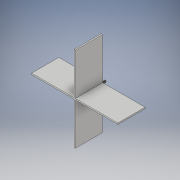
# Autodesk Inventor part: servo part1
Saved by Autodesk Inventor 2019 (Build 230136000, 136)
## iProperties
Created: 2020-02-19
Part Number: servo part1
Material: Generic
Document SubType Name: Modeling
Designer: LENOVO
Density: 1 g/cm^3
Appearance: Default
Author: LENOVO
Autodesk Inventor part; units mm, degrees
ref_plane "YZ Plane" through (0, 0, 0) normal (1, 0, 0) x (0, 1, 0)
ref_plane "XZ Plane" through (0, 0, 0) normal (0, 1, 0) x (-1, 0, 0)
ref_plane "XY Plane" through (0, 0, 0) normal (0, 0, 1) x (1, 0, 0)
sketch "Sketch1" plane through (0, 0, 0) normal (0, 0, 1) x (1, 0, 0)
  circle A0 centre (0, 0) radius 1.5
  dimension "d0" = 3
  constraints: 1 centre point, 1 coincident
  measures "d0" diameter of A0
extrude "Extrusion1" add sketch "Sketch1" along normal blind 4
sketch "Sketch2" plane through (0, 0, 4) normal (0, 0, 1) x (1, 0, 0)
  line L0 (1, 0) -> (-1, 0)
  line L1 (-1, 0) -> (-1, -4)
  line L2 (-1, -4) -> (1, -4)
  line L3 (1, -4) -> (1, 0)
  line L4 (1, 0) -> (-1, 0)
  line L5 (-1, 0) -> (-1, 4)
  line L6 (-1, 4) -> (1, 4)
  line L7 (1, 4) -> (1, 0)
  point P0 (0, 0)
  dimension "d3" = 2
  dimension "d4" = 4
  dimension "d5" = 4
  constraints: 16 end point, 4 parallel, 2 horizontal, 2 perpendicular, 1 point on line
  measures "d3" distance of L2.end L1.end
  measures "d4" distance of L1.end L0.end
  measures "d5" distance of L4.end L5.end
extrude "Extrusion2" add sketch "Sketch2" along normal blind 2
sketch "Sketch3" plane through (0, 0, 4) normal (0, 0, 1) x (1, 0, 0)
  line L0 (1, -4) -> (1, 4) projected
  line L1 (1, 1) -> (5, 1)
  line L2 (5, 1) -> (5, -1)
  line L3 (5, -1) -> (1, -1)
  line L4 (1, -1) -> (1, 1)
  line L5 (-1, 4) -> (-1, -4) projected
  line L6 (-1, 1) -> (-5, 1)
  line L7 (-5, 1) -> (-5, -1)
  line L8 (-5, -1) -> (-1, -1)
  line L9 (-1, -1) -> (-1, 1)
  point P0 (0, 0)
  dimension "d8" = 4
  dimension "d9" = 2
  dimension "d10" = 4
  constraints: 16 end point, 4 parallel, 2 horizontal, 2 perpendicular, 2 point on line
  measures "d8" distance of L2.end L3.end
  measures "d9" distance of L1.end L2.end
  measures "d10" distance of L8.end L7.end
extrude "Extrusion3" add sketch "Sketch3" along normal blind 2
sketch "Sketch4" plane through (0, 0, 4) normal (0, 0, -1) x (-1, 0, 0)
  line L0 (-5, 1) -> (-5, -1) projected
  line L1 (-1.118, 1) -> (-5, 1) projected
  line L2 (-5, -1) -> (-1.5, -1)
  line L3 (-1.5, -1) -> (-1.5, 1)
  line L4 (-1.5, 1) -> (-5, 1)
  line L5 (-5, 1) -> (-5, -1)
  line L6 (1, 4) -> (1, 1.118) projected
  line L7 (-1, 1.118) -> (-1, 4) projected
  line L8 (1, 4) -> (-1, 4)
  line L9 (-1, 4) -> (-1, 1.5)
  line L10 (-1, 1.5) -> (1, 1.5)
  line L11 (1, 1.5) -> (1, 4)
  line L12 (5, -1) -> (1, -1) projected
  line L13 (5, -1) -> (1.5, -1)
  line L14 (1.5, -1) -> (1.5, 1)
  line L15 (1.5, 1) -> (5, 1)
  line L16 (5, 1) -> (5, -1)
  line L17 (1, -1) -> (1, -4) projected
  line L18 (1, -4) -> (-1, -4)
  line L19 (-1, -4) -> (-1, -1.5)
  line L20 (-1, -1.5) -> (1, -1.5)
  line L21 (1, -1.5) -> (1, -4)
  point P0 (0, 0)
  dimension "d13" = 3.5
  dimension "d14" = 2.5
  dimension "d15" = 3.5
  dimension "d16" = 2
  dimension "d17" = 2
  dimension "d18" = 2.5
  constraints: 32 end point, 8 parallel, 4 horizontal, 4 perpendicular, 2 point on line
  measures "d13" distance of L4.end L3.end
  measures "d14" distance of L9.end L8.end
  measures "d15" distance of L14.end L15.end
  measures "d16" distance of L13.end L14.end
  measures "d17" distance of L19.end L20.end
  measures "d18" distance of L18.end L19.end
extrude "Extrusion4" cut sketch "Sketch4" against normal blind 1
sketch "Sketch5" plane through (0, 0, 4) normal (0, 0, -1) x (-1, 0, 0)
  point P0 (0, 0)
fillet "Fillet1" radius 1 8 edges at (-1.5, -1, 4.5) (-1.5, 1, 4.5) (-1, 1.5, 4.5) (1, 1.5, 4.5) (1.5, 1, 4.5) (1.5, -1, 4.5) (1, -1.5, 4.5) (-1, -1.5, 4.5)
sketch "Sketch6" plane through (-5, -1, 6) normal (-1, 0, 0) x (0, 0, 1)
  line L0 (-1, 0.866) -> (-1, 0) projected
  line L1 (0, 2) -> (0, 0) projected
  line L2 (-1, 0) -> (0, 0)
  line L3 (0, 0) -> (0, 2)
  line L4 (0, 2) -> (-1, 2)
  line L5 (-1, 2) -> (-1, 0)
  point P0 (-6, 1)
  constraints: 8 end point, 2 parallel, 1 horizontal, 1 perpendicular
extrude "Extrusion5" add sketch "Sketch6" along normal blind 20
sketch "Sketch7" plane through (-1, -4, 6) normal (0, -1, 0) x (1, 0, 0)
  line L0 (2, -1) -> (1.134, -1) projected
  line L1 (2, -1) -> (0, -1)
  line L2 (0, -1) -> (0, 0)
  line L3 (0, 0) -> (2, 0)
  line L4 (2, 0) -> (2, -1)
  point P0 (1, -6)
  constraints: 8 end point, 2 parallel, 1 horizontal, 1 perpendicular
extrude "Extrusion6" add sketch "Sketch7" along normal blind 20
sketch "Sketch8" plane through (-1, 4, 6) normal (0, 1, 0) x (1, 0, 0)
  line L0 (2, 0) -> (0, 0) projected
  line L1 (0, 1) -> (0, 0) projected
  line L2 (2, 0) -> (0, 0)
  line L3 (0, 0) -> (0, 1)
  line L4 (0, 1) -> (2, 1)
  line L5 (2, 1) -> (2, 0)
  point P0 (1, 6)
  constraints: 8 end point, 2 parallel, 1 horizontal, 1 perpendicular
extrude "Extrusion7" add sketch "Sketch8" along normal blind 20
sketch "Sketch9" plane through (5, -1, 6) normal (1, 0, 0) x (0, 0, -1)
  line L0 (0, 2) -> (1, 2) projected
  line L1 (0, 0) -> (1, 0)
  line L2 (1, 0) -> (1, 2)
  line L3 (1, 2) -> (0, 2)
  line L4 (0, 2) -> (0, 0)
  point P0 (6, 1)
  constraints: 8 end point, 2 parallel, 1 horizontal, 1 perpendicular
extrude "Extrusion8" add sketch "Sketch9" along normal blind 20
sketch "Sketch10" plane through (0, 0, 6) normal (0, 0, 1) x (1, 0, 0)
  line L0 (1, 1) -> (25, 1) projected
  line L1 (-1, -1) -> (-25, -1) projected
  line L2 (25, 1) -> (-25, 1)
  line L3 (-25, 1) -> (-25, -1)
  line L4 (-25, -1) -> (25, -1)
  line L5 (25, -1) -> (25, 1)
  point P0 (0, 0)
  constraints: 8 end point, 2 parallel, 1 horizontal, 1 perpendicular
extrude "Extrusion9" add sketch "Sketch10" along normal blind 20
sketch "Sketch11" plane through (0, 0, 6) normal (0, 0, 1) x (1, 0, 0)
  line L0 (1, -1) -> (1, -24) projected
  line L1 (-1, -1) -> (-1, -24) projected
  line L2 (1, -1) -> (-1, -1)
  line L3 (-1, -1) -> (-1, -24)
  line L4 (-1, -24) -> (1, -24)
  line L5 (1, -24) -> (1, -1)
  arc A0 (-0.134, 1.5) -> (-1, 1) centre (-0.134, 0.5) ccw projected
  line L6 (-1, 24) -> (1, 24) projected
  line L7 (-1, 1) -> (1, 1)
  line L8 (1, 1) -> (1, 24)
  line L9 (1, 24) -> (-1, 24)
  line L10 (-1, 24) -> (-1, 1)
  point P0 (0, 0)
  constraints: 16 end point, 4 parallel, 2 horizontal, 2 perpendicular
extrude "Extrusion10" add sketch "Sketch11" along normal blind 20
sketch "Sketch12" plane through (0, 0, 26) normal (0, 0, 1) x (1, 0, 0)
  line L0 (25, -1) -> (25, 1) projected
  line L1 (-1, -1) -> (-25, -1) projected
  line L2 (25, 1) -> (-25, 1)
  line L3 (-25, 1) -> (-25, -1)
  line L4 (-25, -1) -> (25, -1)
  line L5 (25, -1) -> (25, 1)
  point P0 (0, 0)
  constraints: 8 end point, 2 parallel, 1 horizontal, 1 perpendicular
extrude "Extrusion11" add sketch "Sketch12" along normal blind 20
sketch "Sketch13" plane through (0, 0, 26) normal (0, 0, 1) x (1, 0, 0)
  line L0 (1, 24) -> (-1, 24) projected
  line L1 (-1, 1) -> (1, 1)
  line L2 (1, 1) -> (1, 24)
  line L3 (1, 24) -> (-1, 24)
  line L4 (-1, 24) -> (-1, 1)
  line L5 (1, -24) -> (1, -1) projected
  line L6 (-1, -1) -> (1, -1)
  line L7 (1, -1) -> (1, -24)
  line L8 (1, -24) -> (-1, -24)
  line L9 (-1, -24) -> (-1, -1)
  point P0 (0, 0)
  constraints: 16 end point, 4 parallel, 2 horizontal, 2 perpendicular
extrude "Extrusion12" add sketch "Sketch13" along normal blind 20
sketch "Sketch14" plane through (-1, -24, 6) normal (0, -1, 0) x (1, 0, 0)
  line L0 (0, -1) -> (0, 40) projected
  line L1 (2, -1) -> (2, 40) projected
  line L2 (0, -1) -> (2, -1)
  line L3 (2, -1) -> (2, 40)
  line L4 (2, 40) -> (0, 40)
  line L5 (0, 40) -> (0, -1)
  point P0 (1, -6)
  constraints: 8 end point, 2 parallel, 1 horizontal, 1 perpendicular
extrude "Extrusion13" add sketch "Sketch14" along normal blind 20
sketch "Sketch15" plane through (25, -1, 6) normal (1, 0, 0) x (0, 0, -1)
  line L0 (1, 0) -> (-40, 0) projected
  line L1 (1, 2) -> (-40, 2) projected
  line L2 (1, 0) -> (-40, 0)
  line L3 (-40, 0) -> (-40, 2)
  line L4 (-40, 2) -> (1, 2)
  line L5 (1, 2) -> (1, 0)
  point P0 (6, 1)
  constraints: 8 end point, 2 parallel, 1 horizontal, 1 perpendicular
extrude "Extrusion14" add sketch "Sketch15" along normal blind 20
sketch "Sketch16" plane through (-1, 24, 6) normal (0, 1, 0) x (1, 0, 0)
  line L0 (2.5, 1) -> (2, 1) projected
  line L1 (2, -40) -> (0, -40) projected
  line L2 (2, 1) -> (0, 1)
  line L3 (0, 1) -> (0, -40)
  line L4 (0, -40) -> (2, -40)
  line L5 (2, -40) -> (2, 1)
  point P0 (1, 6)
  constraints: 8 end point, 2 parallel, 1 horizontal, 1 perpendicular
extrude "Extrusion15" add sketch "Sketch16" along normal blind 20
sketch "Sketch17" plane through (-25, -1, 6) normal (-1, 0, 0) x (0, 0, 1)
  line L0 (-1, 0) -> (40, 0) projected
  line L1 (40, 2) -> (40, 0) projected
  line L2 (-1, 0) -> (40, 0)
  line L3 (40, 0) -> (40, 2)
  line L4 (40, 2) -> (-1, 2)
  line L5 (-1, 2) -> (-1, 0)
  point P0 (-6, 1)
  constraints: 8 end point, 2 parallel, 1 horizontal, 1 perpendicular
extrude "Extrusion16" add sketch "Sketch17" along normal blind 20
sketch "Sketch18" plane through (-45, -1, 6) normal (-1, 0, 0) x (0, 0, 1)
  line L0 (40, 2) -> (-1, 2) projected
  line L1 (-1, 0) -> (40, 0)
  line L2 (40, 0) -> (40, 2)
  line L3 (40, 2) -> (-1, 2)
  line L4 (-1, 2) -> (-1, 0)
  point P0 (-6, 1)
  constraints: 8 end point, 2 parallel, 1 horizontal, 1 perpendicular
extrude "Extrusion17" add sketch "Sketch18" along normal blind 20
sketch "Sketch19" plane through (-1, -44, 6) normal (0, -1, 0) x (1, 0, 0)
  line L0 (2, -1) -> (2, -2) projected
  line L1 (0, 40) -> (0, -1) projected
  line L2 (2, -1) -> (0, -1)
  line L3 (0, -1) -> (0, 40)
  line L4 (0, 40) -> (2, 40)
  line L5 (2, 40) -> (2, -1)
  point P0 (1, -6)
  constraints: 8 end point, 2 parallel, 1 horizontal, 1 perpendicular
extrude "Extrusion18" add sketch "Sketch19" along normal blind 20
sketch "Sketch20" plane through (45, -1, 6) normal (1, 0, 0) x (0, 0, -1)
  line L0 (1, 2) -> (1, 1.134) projected
  line L1 (-40, 0) -> (1, 0) projected
  line L2 (1, 2) -> (-40, 2)
  line L3 (-40, 2) -> (-40, 0)
  line L4 (-40, 0) -> (1, 0)
  line L5 (1, 0) -> (1, 2)
  point P0 (6, 1)
  constraints: 8 end point, 2 parallel, 1 horizontal, 1 perpendicular
extrude "Extrusion19" add sketch "Sketch20" along normal blind 20
sketch "Sketch21" plane through (-1, 44, 6) normal (0, 1, 0) x (1, 0, 0)
  line L0 (0, -40) -> (0, 1) projected
  line L1 (2, -40) -> (2, 1) projected
  line L2 (0, 1) -> (2, 1)
  line L3 (2, 1) -> (2, -40)
  line L4 (2, -40) -> (0, -40)
  line L5 (0, -40) -> (0, 1)
  point P0 (1, 6)
  constraints: 8 end point, 2 parallel, 1 horizontal, 1 perpendicular
extrude "Extrusion20" add sketch "Sketch21" along normal blind 20
body "Solid1"
